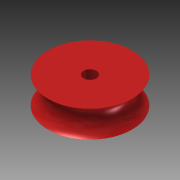
# Autodesk Inventor part: Polea
Saved by Autodesk Inventor 2014 (Build 180170000, 170)
## iProperties
Created: 2016-01-03
Part Number: Polea
Material: Generic
Document SubType Name: Modeling
Designer: Rubén
Density: 1 g/cm^3
Appearance: Light Red
Author: Rubén
Autodesk Inventor part; units mm, degrees
ref_plane "YZ Plane" through (0, 0, 0) normal (1, 0, 0) x (0, 1, 0)
ref_plane "XZ Plane" through (0, 0, 0) normal (0, 1, 0) x (-1, 0, 0)
ref_plane "XY Plane" through (0, 0, 0) normal (0, 0, 1) x (1, 0, 0)
sketch "Sketch1" plane through (0, 0, 0) normal (1, 0, 0) x (0, 1, 0)
  line L0 (0, 0) -> (3.5, 0) construction
  line L1 (3.5, 0) -> (3.5, 1.7) construction
  line L2 (0, 0) -> (0, 13) construction
  arc A0 (0, 8.9689) -> (3.5, 11) centre (0, 13) ccw
  line L3 (0, 0) -> (-3.5, 0) construction
  line L4 (-3.5, 0) -> (-3.5, 1.7) construction
  arc A1 (-3.5, 11) -> (0, 8.9689) centre (0, 13) ccw
  line L5 (-3.5, 1.7) -> (3.5, 1.7)
  line L6 (-3.5, 1.7) -> (-3.5, 11)
  line L7 (3.5, 1.7) -> (3.5, 11)
  dimension "d0" = 7
  dimension "d1" = 13
  dimension "d2" = 1.7
  dimension "d3" = 11
  constraints: 16 end point, 4 perpendicular, 4 point on circle, 2 centre point, 2 parallel, 2 symmetric about line, 1 coincident, 1 horizontal, 1 other
  measures "d0" distance between parallel lines of L1 L4
  measures "d1" distance of L0.start L2.end
  measures "d2" distance between parallel lines of L3 L5
  measures "d3" distance of L0.end L7.end
revolve "Revolution1" add sketch "Sketch1" angle 360 about axis through (0, 0, 0) along (0, 1, 0)
body "Solid1"
